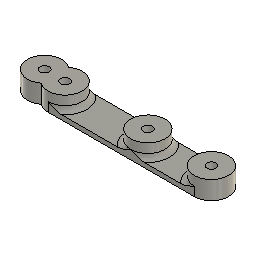
Radio+Rail+Adapter (Autodesk Fusion 360 design; units mm, degrees)
Autodesk Fusion 360 part; units mm, degrees
note: some values were not read from the file. Chosen so that the rebuilt part matches the saved one: which pieces of a blend or face edit are solid.
sketch "bracket main body" plane through (0, 0, 0) normal (0, 0, 1) x (1, 0, 0)
  line L0 (50, 7.5) -> (-50, 7.5)
  line L1 (-50, 7.5) -> (-50, -7.5)
  line L2 (-50, -7.5) -> (50, -7.5)
  line L3 (50, -7.5) -> (50, 7.5)
  line L4 (50, 7.5) -> (-50, -7.5) construction
  line L5 (-50, 7.5) -> (50, -7.5) construction
  dimension "d1" = 100
  dimension "d2" = 15
  constraint horizontal L0
  constraint perpendicular L0 L1
  constraint parallel L0 L2
  constraint parallel L1 L3
  constraint coincident L4 origin
  constraint coincident L5 origin
  measures "d1" distance of L1.end L2.end
  measures "d2" distance of L0.end L1.end
sketch "rail features" plane through (0, 0, 2) normal (0, 0, 1) x (-1, 0, 0)
  line L0 (-50, 7.5) -> (-50, -7.5)
  line L1 (-50, -7.5) -> (50, -7.5)
  line L2 (50, -7.5) -> (50, 7.5)
  line L3 (50, 7.5) -> (-50, 7.5)
  line L4 (50, 0) -> (16, 0) construction
  line L5 (16, 0) -> (-48, 0) construction
  circle A0 centre (16, 0) radius 2
  circle A1 centre (-48, 0) radius 2
  circle A2 centre (16, 0) radius 7.5
  circle A3 centre (-48, 0) radius 7.5
  dimension "d5" = 34
  dimension "d6" = 64
  dimension "d7" = 4
  dimension "d8" = 4
  dimension "d46" = 15
  dimension "d47" = 15
  constraint midpoint L2 L4.start
  constraint perpendicular L2 L4
  constraint parallel L4 L5
  constraint coincident L4.end L5.start
  constraint coincident L5.end A1.centre
  constraint concentric A0 A2
  constraint concentric A1 A3
  measures "d5" distance of L4.start L4.end
  measures "d6" distance of L4.end L5.end
  measures "d7" diameter of A0
  measures "d8" diameter of A1
  measures "d46" diameter of A2
  measures "d47" diameter of A3
sketch "housing features" plane through (0, 0, 0) normal (0, 0, -1) x (1, 0, 0)
  line L0 (50, -7.5) -> (50, 7.5)
  line L1 (50, 7.5) -> (-50, 7.5)
  line L2 (-50, 7.5) -> (-50, -7.5)
  line L3 (-50, -7.5) -> (50, -7.5)
  line L4 (-50, 0) -> (-25, 0) construction
  line L5 (-25, 0) -> (20.2, 0) construction
  circle A0 centre (-25, 0) radius 2
  circle A1 centre (20.2, 0) radius 2
  circle A2 centre (-25, 0) radius 7.5
  circle A3 centre (20.2, 0) radius 7.5
  line L6 (-50, -7.5) -> (-50, 7.5)
  dimension "d19" = 25
  dimension "d20" = 45.2
  dimension "d21" = 4
  dimension "d22" = 4
  dimension "d48" = 15
  dimension "d49" = 15
  dimension "d73" = 50
  constraint midpoint L2 L4.start
  constraint perpendicular L2 L4
  constraint parallel L4 L5
  constraint coincident L4.end L5.start
  constraint coincident L5.end A1.centre
  constraint concentric A0 A2
  constraint concentric A1 A3
  measures "d19" distance of L4.start L4.end
  measures "d20" distance of L4.end L5.end
  measures "d21" diameter of A0
  measures "d22" diameter of A1
  measures "d48" diameter of A2
  measures "d49" diameter of A3
  measures "d73" distance of origin L6
extrude "Extrude6" add sketch "housing features" against normal blind 8 contours A2 makes body 1
extrude "Extrude7" add sketch "housing features" against normal blind 8 separate body contours A3 makes body 2
extrude "Extrude8" add sketch "rail features" along normal blind 6 contours L0 A3 | L0 A3 | A2 bodies 1 makes body 3 at (40.5373, 0.7468, 4)
extrude "Extrude9" add sketch "rail features" against normal blind 2 contours L0 A3 | L0 A3 | L1 L3 A2 A3 | A2 bodies 1 2 3
extrude "Extrude10" cut sketch "housing features" against normal blind 8 contours A0 bodies 1
extrude "Extrude11" cut sketch "rail features" against normal up to surface (8 mm away) from surface at 6 contours A0 bodies 1
fillet "Fillet2" radius 2 1 edges at (-8.5, 0, 2) on bodies 1
fillet "Fillet3" radius 2 1 edges at (27.7, 0, 2) on bodies 1
fillet "Fillet4" radius 2 1 edges at (12.7, 0, 2) on bodies 1
fillet "Fillet5" radius 2 1 edges at (40.5, 0, 2) on bodies 1
extrude "Extrude12" cut 1 faces at (19.5851, 0.0994, 2) along direction (0, 0, -1) blind 2 on bodies 1 bodies 1
equation "d1 = bracketlength"
equation "d2 = bracketheight"
equation "d5 = railoffset"
equation "d6 = railholespace"
equation "d7 = railfastenerclearance"
equation "d8 = railfastenerclearance"
equation "bracketlength = 100 mm"
equation "bracketheight = 15 mm"
equation "bracketthickness = 8 mm"
equation "railoffset = 34 mm"
equation "railthickness = 12.5 mm"
equation "railholespace = 64 mm"
equation "housingoffset = 25 mm"
equation "housingspacing = 45.2 mm"
equation "railfastenerclearance = 4 mm"
equation "housingfastenerclearance = 4 mm"
equation "d19 = housingoffset"
equation "d20 = housingspacing"
equation "d21 = housingfastenerclearance"
equation "d22 = housingfastenerclearance"
equation "bracketbracethickness = 2 mm"
equation "d46 = bracketheight"
equation "d47 = bracketheight"
equation "d48 = bracketheight"
equation "d49 = bracketheight"
equation "d50 = -bracketthickness"
equation "d52 = -bracketthickness"
